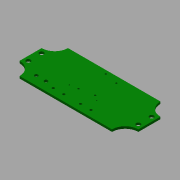
# Autodesk Inventor part: pcb
Saved by Autodesk Inventor 2013 (Build 170138000, 138)
## iProperties
Created: 2014-06-07
Part Number: pcb
Material: Generic
Document SubType Name: Modeling
Designer: Brad
Density: 1 g/cm^3
Author: Brad
Autodesk Inventor part; units mm, degrees
ref_plane "YZ Plane" through (0, 0, 0) normal (1, 0, 0) x (0, 1, 0)
ref_plane "XZ Plane" through (0, 0, 0) normal (0, 1, 0) x (-1, 0, 0)
ref_plane "XY Plane" through (0, 0, 0) normal (0, 0, 1) x (1, 0, 0)
sketch "Sketch1" plane through (0, 0, 0) normal (0, 1, 0) x (-1, 0, 0)
  line L0 (-33.3375, 17.4625) -> (33.3375, 17.4625)
  line L1 (42.8625, 7.9375) -> (42.8625, -7.9375)
  line L2 (33.3375, -17.4625) -> (-33.3375, -17.4625)
  line L3 (-42.8625, -7.9375) -> (-42.8625, 7.9375)
  arc A0 (-42.8625, 7.9375) -> (-33.3375, 17.4625) centre (-42.8625, 17.4625) ccw
  arc A1 (-33.3375, -17.4625) -> (-42.8625, -7.9375) centre (-42.8625, -17.4625) ccw
  arc A2 (42.8625, -7.9375) -> (33.3375, -17.4625) centre (42.8625, -17.4625) ccw
  arc A3 (33.3375, 17.4625) -> (42.8625, 7.9375) centre (42.8625, 17.4625) ccw
  circle A4 centre (-39.6875, -4.7625) radius 1.5875
  line L4 (0, 15.213) -> (0, -8.9791)
  circle A5 centre (39.6875, -4.7625) radius 1.5875
  line L5 (-13.6455, 0) -> (11.519, 0)
  circle A6 centre (-39.6875, 4.7625) radius 1.5875
  circle A7 centre (39.6875, 4.7625) radius 1.5875
  line L6 (-42.8625, -13.6689) -> (-42.8625, -17.4625)
  line L7 (-42.8625, -17.4625) -> (-40.918, -17.4625)
  circle A8 centre (6.0427, 12.8524) radius 0.9004
  circle A9 centre (13.6423, 12.8524) radius 0.9004
  circle A10 centre (-6.0427, 12.8524) radius 0.9004
  circle A11 centre (-13.6423, 12.8524) radius 0.9004
  circle A12 centre (20.6375, 11.1125) radius 1.27
  circle A13 centre (27.6225, 11.1125) radius 1.27
  circle A14 centre (-9.8425, 5.0546) radius 0.4001
  circle A15 centre (9.8425, 5.0546) radius 0.4001
  circle A16 centre (4.13, 4.1021) radius 0.6502
  circle A17 centre (-6.0198, -12.9972) radius 0.6502
  circle A18 centre (-6.0198, 2.2022) radius 0.6502
  circle A19 centre (3.4798, -14.8971) radius 0.6502
  line L8 (-13.6423, 12.8524) -> (-6.0427, 12.8524)
  point P0 (0, 0)
  dimension "d3" = 17.4625
  dimension "d4" = 42.8625
  dimension "d5" = 19.05
  dimension "d6" = 19.05
  dimension "d7" = 19.05
  dimension "d8" = 19.05
  dimension "d9" = 85.725
  dimension "d11" = 85.725
  dimension "d12" = 85.725
  dimension "d13" = 17.4625
  dimension "d14" = 17.4625
  dimension "d15" = 42.8625
  dimension "d19" = 34.925
  dimension "d20" = 42.8625
  dimension "d22" = 17.4625
  dimension "d23" = 42.8625
  dimension "d26" = 39.6875
  dimension "d27" = 3.175
  dimension "d28" = 4.7625
  dimension "d29" = 42.8625
  dimension "d30" = 17.4625
  dimension "d31" = 42.8625
  dimension "d32" = 34.925
  dimension "d33" = 1.8009
  dimension "d34" = 48.9052
  dimension "d35" = 30.3149
  dimension "d36" = 1.8009
  dimension "d37" = 1.8009
  dimension "d38" = 1.8009
  dimension "d39" = 30.3149
  dimension "d40" = 30.3149
  dimension "d41" = 30.3149
  dimension "d42" = 29.2202
  dimension "d43" = 36.8198
  dimension "d45" = 6.0427
  dimension "d46" = 6.0427
  dimension "d47" = 2.54
  dimension "d48" = 2.54
  dimension "d49" = 63.5
  dimension "d50" = 70.485
  dimension "d51" = 28.575
  dimension "d52" = 28.575
  dimension "d53" = 0.8001
  dimension "d54" = 0.8001
  dimension "d55" = 33.02
  dimension "d56" = 52.705
  dimension "d57" = 22.5171
  dimension "d58" = 22.5171
  dimension "d59" = 1.3005
  dimension "d60" = 46.3423
  dimension "d61" = 21.5646
  dimension "d62" = 1.3005
  dimension "d63" = 1.3005
  dimension "d64" = 1.3005
  dimension "d65" = 36.8427
  dimension "d66" = 19.6647
  dimension "d67" = 36.8427
  dimension "d68" = 4.4653
  dimension "d69" = 46.3423
  dimension "d70" = 2.5654
  dimension "d73" = 56.5048
  dimension "d74" = 7.5997
  dimension "d75" = 7.5997
  dimension "d76" = 19.685
  constraints: 20 centre point, 18 end point, 8 point on circle, 4 perpendicular, 3 parallel, 3 symmetric about line, 1 horizontal, 3 other
  measures "d3" distance from line of point (0, 0) L0
  measures "d4" distance from line of point (0, 0) L1
  measures "d5" diameter of A0
  measures "d6" diameter of A1
  measures "d7" diameter of A2
  measures "d8" diameter of A3
  measures "d9" distance between parallel lines of L1 L3
  measures "d11" distance of A0.centre A3.centre
  measures "d12" distance of A1.centre A2.centre
  measures "d13" vertical distance of point (0, 0) A2.centre
  measures "d14" vertical distance of A1.centre point (0, 0)
  measures "d15" horizontal distance of point (0, 0) A1.centre
  measures "d19" distance between parallel lines of L2 L0
  measures "d20" horizontal distance of point (0, 0) A3.centre
  measures "d22" vertical distance of point (0, 0) A3.centre
  measures "d23" horizontal distance of point (0, 0) A0.centre
  measures "d26" horizontal distance of A4.centre point (0, 0)
  measures "d27" diameter of A4
  measures "d28" vertical distance of point (0, 0) A4.centre
  measures "d29" distance between parallel lines of L3 L4
  measures "d30" distance between parallel lines of L2 L5
  measures "d31" distance between parallel lines of L4 L6
  measures "d32" distance between parallel lines of L0 L7
  measures "d33" diameter of A8
  measures "d34" distance from line of L3 A8.centre
  measures "d35" distance from line of L2 A8.centre
  measures "d36" diameter of A9
  measures "d37" diameter of A10
  measures "d38" diameter of A11
  measures "d39" distance from line of L2 L8.start
  measures "d40" distance from line of L2 L8.end
  measures "d41" distance from line of L2 A9.centre
  measures "d42" distance from line of L3 L8.start
  measures "d43" distance from line of L3 L8.end
  measures "d45" distance from line of L4 A8.centre
  measures "d46" distance from line of L8.end L4
  measures "d47" diameter of A12
  measures "d48" diameter of A13
  measures "d49" distance from line of L3 A12.centre
  measures "d50" distance from line of L3 A13.centre
  measures "d51" distance from line of L2 A12.centre
  measures "d52" distance from line of L2 A13.centre
  measures "d53" diameter of A14
  measures "d54" diameter of A15
  measures "d55" distance from line of L3 A14.centre
  measures "d56" distance from line of L3 A15.centre
  measures "d57" distance from line of L2 A14.centre
  measures "d58" distance from line of L2 A15.centre
  measures "d59" diameter of A16
  measures "d60" distance edge to line of A16 L3
  measures "d61" distance from line of L2 A16.centre
  measures "d62" diameter of A17
  measures "d63" diameter of A18
  measures "d64" diameter of A19
  measures "d65" distance from line of L3 A18.centre
  measures "d66" distance from line of L2 A18.centre
  measures "d67" distance from line of A17.centre L3
  measures "d68" distance from line of L2 A17.centre
  measures "d69" distance from line of L3 A19.centre
  measures "d70" distance from line of L2 A19.centre
  measures "d73" distance from line of L3 A9.centre
  measures "d74" distance of L8.end L8.start
  measures "d75" distance of A9.centre A8.centre
  measures "d76" distance of A9.centre L8.end
extrude "Extrusion2" add sketch "Sketch1" along normal blind 1.5748
body "Solid2"
